hole (Autodesk Fusion 360 design; units mm, degrees)
part number: 2026-06-12-02-40-01-817
Autodesk Fusion 360 part; units mm, degrees
sketch "Sketch1" plane through (0, 0, 0) normal (0, 1, 0) x (1, 0, 0)
  circle A0 centre (0, 0) radius 33.0715
  circle A1 centre (0, 0) radius 22
  dimension "d1" = 66.143
  dimension "d2" = 44
  constraint coincident A0.centre A1.centre
  constraint concentric A0 A1
  measures "d1" diameter of A0
  measures "d2" diameter of A1
extrude "Extrude1" add sketch "Sketch1" along normal blind 3
